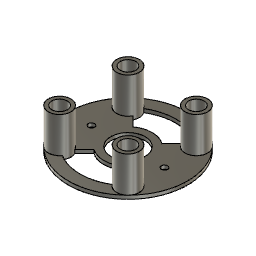
Servo block R5 v10 (Autodesk Fusion 360 archive; units mm, degrees)
design "Magnet attach R3"
Autodesk Fusion 360 part; units mm, degrees
note: some values were not read from the file. Set by a fixed rule: which face or edge a step refers to.
sketch "Sketch1" plane through (0, 0, 0) normal (0, 0, 1) x (1, 0, 0)
  circle A0 centre (0, 0) radius 25.3 construction
  circle A1 centre (0, 0) radius 25.1
  circle A2 centre (0, 0) radius 23.6
  circle A3 centre (0, 0) radius 20.1
  circle A4 centre (0, 0) radius 7.2
  circle A5 centre (0, 0) radius 10.2
  line L0 (0, 0) -> (10.2, 0) construction
  line L1 (0, 0) -> (0, 10.2) construction
  line L2 (0, 0) -> (17.8898, 17.8898) construction
  line L3 (1.0607, -1.0607) -> (18.9505, 16.8291)
  line L4 (-1.0607, 1.0607) -> (16.8291, 18.9505)
  line L5 (-1.0607, 1.0607) -> (1.0607, -1.0607)
  line L6 (-1.0607, -1.0607) -> (-18.9505, 16.8291)
  line L7 (-1.0607, -1.0607) -> (1.0607, 1.0607)
  line L8 (1.0607, 1.0607) -> (-16.8291, 18.9505)
  line L9 (1.0607, -1.0607) -> (-16.8291, -18.9505)
  line L10 (1.0607, -1.0607) -> (-1.0607, 1.0607)
  line L11 (-1.0607, 1.0607) -> (-18.9505, -16.8291)
  line L12 (1.0607, 1.0607) -> (18.9505, -16.8291)
  line L13 (1.0607, 1.0607) -> (-1.0607, -1.0607)
  line L14 (-1.0607, -1.0607) -> (16.8291, -18.9505)
  dimension "d1" = 50.6
  dimension "d4" = 1.5
  dimension "d5" = 5
  dimension "d6" = 14.4
  dimension "d11" = 3
  dimension "d29" = -0.2
  dimension "d31" = 45
  dimension "d32" = 1.5
  dimension "d33" = -1.5
  dimension "d35" = 360
  constraint coincident A0.centre A1.centre
  constraint concentric A0 A2
  constraint concentric A2 A3
  constraint coincident A5 L0.end
  constraint horizontal L0
  constraint coincident A5 L1.end
  constraint perpendicular L0 L1
  constraint coincident A0 L2.end
  constraint perpendicular L3 L5
  measures "d1" diameter of A0
  measures "d4" distance of A1 A2
  measures "d5" distance of A1 A3
  measures "d6" diameter of A4
  measures "d31" angle of L0 L2
extrude "Extrude1" add sketch "Sketch1" along normal blind 1.5 contours A1 A2 L3 L12 | A1 A2 L3 L4 | A1 A2 L12 L14 | A1 A2 L4 L8 | A2 A3 L3 L4 | A2 A3 L3 L12 | A1 A2 L9 L14 | A2 A3 L12 L14 | A1 A2 L6 L8 | A2 A3 L4 L8 | A3 A5 L3 L4 | A1 A2 L9 L11 | A2 A3 L9 L14 | A3 A5 L12 L14 | A1 A2 L6 L11 | A2 A3 L6 L8 | A4 A5 L3 L4 | A4 A5 L3 L12 | A2 A3 L9 L11 | A4 A5 L12 L14 | A2 A3 L6 L11 | A3 A5 L6 L8 | A4 A5 L4 L8 | A3 A5 L9 L11 | A4 A5 L9 L14 | A4 A5 L6 L8 | A4 A5 L9 L11 | A4 A5 L6 L11
sketch "Sketch2" plane through (0, 0, 0) normal (0, 0, 1) x (1, 0, 0)
  circle A0 centre (0, 0) radius 25.1
  line L0 (0, 0) -> (0, 25.1) construction
  circle A1 centre (0, 25.1) radius 1
  dimension "d14" = 2
  constraint coincident A0.centre L0.start
  constraint coincident A0 L0.end
  constraint vertical L0
  constraint coincident L0.end A1.centre
  measures "d14" diameter of A1
ref_plane "WorkPlane1" through (0, 0, 1.5) normal (0, 0, 1) x (1, 0, 0)
sketch "Sketch3" plane through (0, 0, 1.5) normal (0, 0, 1) x (1, 0, 0)
  circle A0 centre (0, 0) radius 25.1 construction
  line L0 (0, 0) -> (0, 25.1) construction
  circle A1 centre (14.3896, 14.3896) radius 3.25
  circle A2 centre (14.3896, 14.3896) radius 4.75
  line L1 (14.3896, 14.3896) -> (14.3896, 19.1396) construction
  line L2 (0, 0) -> (-25.1, 0) construction
  circle A3 centre (-14.3896, 14.3896) radius 4.75
  circle A4 centre (-14.3896, 14.3896) radius 3.25
  line L3 (0, 0) -> (0, -25.1) construction
  circle A5 centre (-14.3896, -14.3896) radius 4.75
  circle A6 centre (-14.3896, -14.3896) radius 3.25
  line L4 (0, 0) -> (25.1, 0) construction
  circle A7 centre (14.3896, -14.3896) radius 4.75
  circle A8 centre (14.3896, -14.3896) radius 3.25
  line L5 (0, 0) -> (17.7484, 17.7484) construction
  line L6 (17.7484, 17.7484) -> (23.1719, 12.3249) construction
  line L7 (14.3896, 14.3896) -> (17.7484, 17.7484) construction
  line L8 (17.7484, 17.7484) -> (26.4317, 9.0651) construction
  arc A9 (15.2339, -13.1126) -> (15.2339, 13.1126) centre (0, 0) ccw
  line L9 (15.2339, -13.1126) -> (8.1947, -6.0734)
  line L10 (8.1947, 6.0734) -> (15.2339, 13.1126)
  line L11 (13.1126, 15.2339) -> (6.0734, 8.1947)
  line L12 (-6.0734, 8.1947) -> (-13.1126, 15.2339)
  arc A10 (13.1126, 15.2339) -> (-13.1126, 15.2339) centre (0, 0) ccw
  line L13 (-13.1126, -15.2339) -> (-6.0734, -8.1947)
  line L14 (6.0734, -8.1947) -> (13.1126, -15.2339)
  arc A11 (-13.1126, -15.2339) -> (13.1126, -15.2339) centre (0, 0) ccw
  line L15 (-15.2339, 13.1126) -> (-8.1947, 6.0734)
  line L16 (-8.1947, -6.0734) -> (-15.2339, -13.1126)
  arc A12 (-15.2339, 13.1126) -> (-15.2339, -13.1126) centre (0, 0) ccw
  arc A13 (-8.1947, 6.0734) -> (-8.1947, -6.0734) centre (0, 0) ccw
  arc A14 (6.0734, 8.1947) -> (-6.0734, 8.1947) centre (0, 0) ccw
  arc A15 (8.1947, -6.0734) -> (8.1947, 6.0734) centre (0, 0) ccw
  arc A16 (-6.0734, -8.1947) -> (6.0734, -8.1947) centre (0, 0) ccw
  circle A17 centre (0, 0) radius 7.2
  circle A18 centre (0, 0) radius 25.1
  dimension "d20" = 6.5
  dimension "d21" = 1.5
  dimension "d23" = 360
  dimension "d30" = 45
  constraint concentric A0 A18
  constraint coincident A0.centre L0.start
  constraint coincident A0 L0.end
  constraint coincident A1.centre A2.centre
  constraint coincident A2 L1.end
  constraint parallel L0 L1
  constraint perpendicular L5 L6
  constraint coincident A1.centre L5
  constraint parallel L5 L7
  constraint coincident A2 L5.end
  constraint tangent A2 L8
  constraint collinear L6 L8
  measures "d20" diameter of A1
  measures "d30" angle of L4 L5
extrude "Extrude3" add sketch "Sketch3" along normal blind 15 contours A1 A2 A9 A10 | A1 A2 L11 A10 | A1 A2 A9 L10 | A1 A2 L10 L11 | A3 A4 A10 A12 | A3 A4 L12 A10 | A7 A8 A9 L9 | A7 A8 A9 A11 | A7 A8 L9 L14 | A3 A4 L15 A12 | A5 A6 A11 A12 | A3 A4 L12 L15 | A7 A8 L14 A11 | A5 A6 L16 A12 | A5 A6 L13 A11 | A5 A6 L13 L16
extrude "Extrude4" add sketch "Sketch3" against normal up to surface (1.5 mm away) contours A1 A9 L10 L11 A10 | A1 A2 A9 A10 | A1 L11 A10 | A1 A2 L11 A10 | A1 A2 A9 L10 | A1 A9 L10 | A1 A2 L10 L11 | A3 A4 A10 A12 | A3 A4 L12 A10 | A7 A8 A9 L9 | A7 A8 A9 A11 | A4 L12 A10 L15 A12 | A4 L12 A10 | A7 A8 L9 L14 | A8 A9 L9 | A8 A9 L9 L14 A11 | A3 A4 L15 A12 | A5 A6 A11 A12 | A3 A4 L12 L15 | A4 L15 A12 | A7 A8 L14 A11 | A5 A6 L16 A12 | A5 A6 L13 A11 | A8 L14 A11 | A5 A6 L13 L16 | A6 L13 A11 L16 A12 | A6 L16 A12 | A6 L13 A11
ref_plane "WorkPlane3" through (0, 0, 1.5) normal (0, 0, 1) x (1, 0, 0)
sketch "Sketch5" plane through (0, 0, 1.5) normal (0, 0, 1) x (1, 0, 0)
  circle A0 centre (-14.3896, 14.3896) radius 3.25
  circle A1 centre (-14.3896, 14.3896) radius 4.75
  circle A2 centre (14.3896, 14.3896) radius 3.25
  circle A3 centre (14.3896, 14.3896) radius 4.75
  circle A4 centre (14.3896, -14.3896) radius 3.25
  circle A5 centre (14.3896, -14.3896) radius 4.75
  circle A6 centre (-14.3896, -14.3896) radius 3.25
  circle A7 centre (-14.3896, -14.3896) radius 4.75
  line L0 (-15.35, 20) -> (15.35, 20) construction
  line L1 (15.35, 20) -> (15.35, -20) construction
  line L2 (15.35, -20) -> (-15.35, -20) construction
  line L3 (-15.35, -20) -> (-15.35, 20) construction
  line L4 (0, 20) -> (0, -20) construction
  line L5 (-15.35, 0) -> (15.35, 0) construction
  line L6 (-28.2065, 6) -> (30.7422, 6)
  line L7 (-28.663, -6) -> (31.8265, -6)
  arc A8 (-8.1947, 6.0734) -> (-8.1947, -6.0734) centre (0, 0) ccw
  arc A9 (8.1947, -6.0734) -> (8.1947, 6.0734) centre (0, 0) ccw
  arc A10 (17.1324, -10.5115) -> (17.1324, 10.5115) centre (0, 0) ccw
  arc A11 (-17.1324, 10.5115) -> (-17.1324, -10.5115) centre (0, 0) ccw
  line L8 (-12.2634, 10.1421) -> (-8.1947, 6.0734)
  line L9 (8.1947, 6.0734) -> (12.2634, 10.1421)
  line L10 (12.2634, -10.1421) -> (8.1947, -6.0734)
  line L11 (-8.1947, -6.0734) -> (-12.2634, -10.1421)
  circle A12 centre (-15.35, 0) radius 1.325
  circle A13 centre (15.35, 0) radius 1.325
  dimension "d52" = 40
  dimension "d53" = 30.7
  dimension "d71" = 6
  dimension "d72" = 6
  dimension "d74" = 2.65
  dimension "d75" = 2.65
  constraint horizontal L0
  constraint vertical L1
  constraint horizontal L2
  constraint vertical L3
  constraint midpoint L0 L4.start
  constraint midpoint L2 L4.end
  constraint midpoint L3 L5.start
  constraint midpoint L1 L5.end
  constraint coincident A8.centre L4
  constraint coincident A8.centre L5
  constraint horizontal L6
  constraint perpendicular L3 L7
  constraint coincident L5.start A12.centre
  constraint coincident L5.end A13.centre
  measures "d52" distance of L0.end L1.end
  measures "d53" distance of L0.start L0.end
  measures "d71" distance of L5 L7
  measures "d72" distance of L5 L6
  measures "d74" diameter of A12
  measures "d75" diameter of A13
extrude "Extrude5" cut sketch "Sketch3" against normal up to surface (1.5 mm away) contours A1 A9 L10 L11 A10 | A1 L11 A10 | A1 A9 L10 | A4 L12 A10 L15 A12 | A4 L12 A10 | A8 A9 L9 | A8 A9 L9 L14 A11 | A4 L15 A12 | A8 L14 A11 | A6 L13 A11 L16 A12 | A6 L16 A12 | A6 L13 A11
extrude "Extrude7" add sketch "Sketch5" against normal up to surface (1.5 mm away) contours A0 | A1 L6 A8 A11 L8 | L6 L7 A8 A11 | A7 L7 A8 A11 L11 | A3 L6 A9 A10 L9 | L6 L7 A9 A10 | A5 L7 A9 A10 L10 | A2 | A4 | A6
ref_plane "WorkPlane4" through (0, 0, 1.5) normal (0, 0, 1) x (1, 0, 0)
extrude "Extrude8" add sketch "Sketch3" along normal blind 5 contours A1 A9 L10 L11 A10 | A1 L11 A10 | A1 A9 L10 | A4 L12 A10 L15 A12 | A4 L12 A10 | A8 A9 L9 | A8 A9 L9 L14 A11 | A4 L15 A12 | A8 L14 A11 | A6 L13 A11 L16 A12 | A6 L16 A12 | A6 L13 A11
equation "k = 0.4 mm"
equation "d20 = 6 mm + 0.6 mm - 0.1 mm"
equation "d53 = ( 15.35 * 2 ) * 1 mm"
equation "mag = 6.35 mm + 0.5 mm"
equation "mag_depth = 3.175 mm + 0.6 mm"
equation "screw = 2.35 mm + 0.3 mm"
equation "d74 = screw"
equation "d75 = screw"
equation "d55 = mag"
equation "d57 = mag"
equation "d67 = mag_depth"

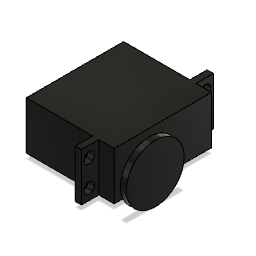
design "HS-311"
Autodesk Fusion 360 part; units mm, degrees
sketch "Sketch1" plane through (0, 0, 0) normal (0, 0, 1) x (1, 0, 0) in component "MG995 v1 (1)"
  line L0 (-20.2, 9.95) -> (20.2, 9.95)
  line L1 (20.2, 9.95) -> (20.2, -9.95)
  line L2 (20.2, -9.95) -> (-20.2, -9.95)
  line L3 (-20.2, -9.95) -> (-20.2, 9.95)
  line L4 (0, 9.95) -> (0, -9.95) construction
  line L5 (-20.2, 0) -> (20.2, 0) construction
  dimension "d1_1_1_1_1" = 40.4
  dimension "d2_1_1_1_1" = 19.9
  constraint horizontal L0
  constraint vertical L1
  constraint horizontal L2
  constraint vertical L3
  constraint midpoint L0 L4.start
  constraint midpoint L2 L4.end
  constraint midpoint L3 L5.start
  constraint midpoint L1 L5.end
  constraint coincident origin L5
  constraint coincident origin L4
  measures "d1_1_1_1_1" distance of L0.start L0.end
  measures "d2_1_1_1_1" distance of L0.start L2.end
extrude "Extrude1" add sketch "Sketch1" along normal blind 36.5 in component "MG995 v1 (1)"
sketch "Sketch2" plane through (0, 0, 36.5) normal (0, 0, 1) x (1, 0, 0) in component "MG995 v1 (1)"
  line L0 (-20.2, -9.95) -> (20.2, -9.95)
  line L1 (20.2, -9.95) -> (20.2, 9.95)
  line L2 (20.2, 9.95) -> (-20.2, 9.95)
  line L3 (-20.2, 9.95) -> (-20.2, -9.95)
  line L4 (20.2, 9.95) -> (-20.2, 9.95)
  line L5 (-20.2, -9.95) -> (20.2, -9.95)
  line L6 (-10.7, 9.95) -> (-10.7, -9.95) construction
  circle A0 centre (-10.7, 0) radius 2.9
  line L7 (0, 9.95) -> (0, -9.95) construction
  dimension "d5_1_1_1_1" = 5.8
  dimension "d8_1_1_1_1" = 9.5
  constraint coincident L2 L6.start
  constraint coincident L0 L6.end
  constraint perpendicular L0 L6
  constraint midpoint L6 A0.centre
  constraint midpoint L4 L7.start
  constraint midpoint L5 L7.end
  measures "d5_1_1_1_1" diameter of A0
  measures "d8_1_1_1_1" distance of L3 L6
extrude "Extrude2" add sketch "Sketch2" along normal blind 5.06 contours A0 in component "MG995 v1 (1)"
ref_plane "WorkPlane1" through (0, 0, 27.5) normal (0, 0, -1) x (-1, 0, 0) in component "MG995 v1 (1)"
sketch "Sketch3" plane through (-4.1411, 18.8966, 27.5) normal (0, 0, -1) x (1, 0, 0) in component "MG995 v1 (1)"
  line L0 (31.5411, 8.9466) -> (-23.2589, 8.9466)
  line L1 (-23.2589, 8.9466) -> (-23.2589, 28.8466)
  line L2 (-23.2589, 28.8466) -> (31.5411, 28.8466)
  line L3 (31.5411, 28.8466) -> (31.5411, 8.9466)
  line L4 (24.3411, 28.8466) -> (-16.0589, 28.8466)
  line L5 (-16.0589, 8.9466) -> (24.3411, 8.9466)
  line L6 (24.3411, 8.9466) -> (24.3411, 28.8466)
  line L7 (-16.0589, 28.8466) -> (-16.0589, 8.9466)
  circle A0 centre (28.3411, 13.4466) radius 2.2
  circle A1 centre (28.3411, 24.3466) radius 2.2
  circle A2 centre (-20.0589, 13.4466) radius 2.2
  circle A3 centre (-20.0589, 24.3466) radius 2.2
  line L8 (28.3411, 8.9466) -> (28.3411, 28.8466) construction
  line L9 (-20.0589, 8.9466) -> (-20.0589, 28.8466) construction
  dimension "d10_1_1_1_1" = 7.2
  dimension "d11_1_1_1_1" = 7.2
  dimension "d12_1_1_1_1" = 4.4
  dimension "d13_1_1_1" = 4.4
  dimension "d14_1_1_1" = 4.4
  dimension "d15_1_1_1" = 4.4
  dimension "d16_1_1_1" = 4.5
  dimension "d17_1_1_1" = 4.5
  dimension "d18_1_1_1" = 4.5
  dimension "d19_1_1_1" = 4.5
  dimension "d20_1_1_1" = 3.2
  dimension "d21_1_1_1" = 3.2
  constraint horizontal L0
  constraint vertical L1
  constraint horizontal L2
  constraint vertical L3
  constraint collinear L2 L4
  constraint collinear L0 L5
  constraint coincident L0 L8.start
  constraint coincident L2 L8.end
  constraint perpendicular L2 L8
  constraint coincident L0 L9.start
  constraint coincident L2 L9.end
  constraint perpendicular L2 L9
  constraint coincident A0.centre L8
  constraint coincident A1.centre L8
  constraint coincident A2.centre L9
  constraint coincident A3.centre L9
  measures "d10_1_1_1_1" distance of L3 L6
  measures "d11_1_1_1_1" distance of L1 L7
  measures "d12_1_1_1_1" diameter of A0
  measures "d13_1_1_1" diameter of A1
  measures "d14_1_1_1" diameter of A2
  measures "d15_1_1_1" diameter of A3
  measures "d16_1_1_1" distance of L0 A0.centre
  measures "d17_1_1_1" distance of L2 A1.centre
  measures "d18_1_1_1" distance of L0 A2.centre
  measures "d19_1_1_1" distance of L2 A3.centre
  measures "d20_1_1_1" distance of L3 L8
  measures "d21_1_1_1" distance of L1 L9
extrude "Extrude3" add sketch "Sketch3" against normal blind 2.6 contours L0 L2 L3 L6 | L0 L1 L2 L7 in component "MG995 v1 (1)"
sketch "Sketch5" plane through (0, 0, 41.56) normal (0, 0, 1) x (1, 0, 0) in component "MG995 v1 (1)"
  circle A0 centre (-10.7, 0) radius 2.9
  circle A1 centre (-10.7, 0) radius 11.98
  dimension "d494_1_1_1" = 23.96
  constraint concentric A0 A1
  measures "d494_1_1_1" diameter of A1
extrude "Extrude5" add sketch "Sketch5" along normal blind 2.5 contours A0 | A1 in component "MG995 v1 (1)"
component "MG995 v1 (1)" placed x (0, 1, 0) y (0, 0, 1) z (1, 0, 0) at (-69.2471, 31.7306, -29.2908)
